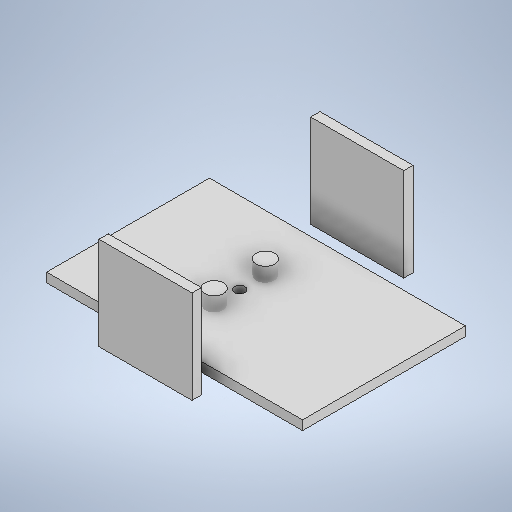
# Autodesk Inventor part: Rahmen_v4
Saved by Autodesk Inventor 2025 (Build 290162000, 162)
## iProperties
Created: 2026-07-01
Part Number: Rahmen_v4
Material: Generisch
Document SubType Name: Modeling
Designer: wavid
Density: 1 g/cm^3
Appearance: Vorgabe
Author: wavid
Autodesk Inventor part; units mm, degrees
sketch "Skizze1" plane through (0, 0, 0) normal (0, 0, 1) x (1, 0, 0)
  line L0 (-110, -70) -> (110, -70)
  line L1 (110, -70) -> (110, 70)
  line L2 (110, 70) -> (-110, 70)
  line L3 (-110, 70) -> (-110, -70)
  constraints: 8 end point, 2 parallel, 1 horizontal, 1 perpendicular
extrude "Extrusion1" add sketch "Skizze1" along normal blind 8
sketch "Skizze2" plane through (0, 0, 0) normal (0, 0, 1) x (1, 0, 0)
  circle A0 centre (-14, -22) radius 8
  constraints: 1 centre point
extrude "Extrusion2" add sketch "Skizze2" along normal blind 20 separate body
sketch "Skizze3" plane through (0, 0, 0) normal (0, 0, 1) x (1, 0, 0)
  circle A0 centre (-14, 22) radius 8
  constraints: 1 centre point
extrude "Extrusion3" add sketch "Skizze3" along normal blind 20 separate body
sketch "Skizze4" plane through (0, 0, 0) normal (0, 0, 1) x (1, 0, 0)
  line L0 (-40, -95) -> (40, -95)
  line L1 (40, -95) -> (40, -87)
  line L2 (40, -87) -> (-40, -87)
  line L3 (-40, -87) -> (-40, -95)
  constraints: 8 end point, 2 parallel, 1 horizontal, 1 perpendicular
extrude "Extrusion4" add sketch "Skizze4" along normal blind 80 separate body
sketch "Skizze5" plane through (0, 0, 0) normal (0, 0, 1) x (1, 0, 0)
  line L0 (-40, 87) -> (40, 87)
  line L1 (40, 87) -> (40, 95)
  line L2 (40, 95) -> (-40, 95)
  line L3 (-40, 95) -> (-40, 87)
  constraints: 8 end point, 2 parallel, 1 horizontal, 1 perpendicular
extrude "Extrusion5" add sketch "Skizze5" along normal blind 80 separate body
ref_plane "Arbeitsebene1" through (0, 0, 20) normal (0, 0, 1) x (1, 0, 0)
ref_plane "Arbeitsebene2" through (0, 0, 8) normal (0, 0, 1) x (1, 0, 0)
sketch "Skizze6" plane through (0, 0, 20) normal (0, 0, 1) x (1, 0, 0)
  circle A0 centre (-14, -22) radius 3.9
  constraints: 1 centre point
extrude "Extrusion6" cut sketch "Skizze6" against normal blind 16 bodies 1
sketch "Skizze7" plane through (0, 0, 20) normal (0, 0, 1) x (1, 0, 0)
  circle A0 centre (-14, 22) radius 3.9
  constraints: 1 centre point
extrude "Extrusion7" cut sketch "Skizze7" against normal blind 16 bodies 1
sketch "Skizze8" plane through (0, 0, 8) normal (0, 0, 1) x (1, 0, 0)
  circle A0 centre (-14, 0) radius 4.5
  constraints: 1 centre point
extrude "Extrusion8" cut sketch "Skizze8" against normal blind 9 bodies 1
ref_plane "Arbeitsebene3" through (0, -91, 0) normal (0, 1, 0) x (-1, 0, 0)
sketch "Skizze9" plane through (0, -91, 0) normal (0, 1, 0) x (-1, 0, 0)
  circle A0 centre (0, 60) radius 7
  constraints: 1 centre point
extrude "Extrusion9" cut sketch "Skizze9" along normal mid plane 12 bodies 1
sketch "Skizze10" plane through (0, -91, 0) normal (0, 1, 0) x (-1, 0, 0)
  circle A0 centre (16, 60) radius 1.5
  constraints: 1 centre point
extrude "Extrusion10" cut sketch "Skizze10" along normal mid plane 12 bodies 1
ref_plane "Arbeitsebene4" through (0, 91, 0) normal (0, 1, 0) x (-1, 0, 0)
sketch "Skizze11" plane through (0, 91, 0) normal (0, 1, 0) x (-1, 0, 0)
  circle A0 centre (0, 60) radius 4.15
  constraints: 1 centre point
extrude "Extrusion11" cut sketch "Skizze11" along normal mid plane 12 bodies 1
